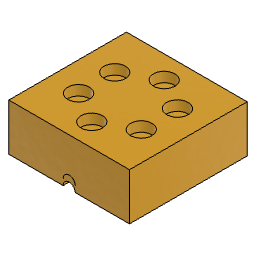
Tool change - six magnets (Autodesk Fusion 360 design; units mm, degrees)
Autodesk Fusion 360 part; units mm, degrees
note: some values were not read from the file. Set by a fixed rule: which sketch regions a step uses.
sketch "Sketch1" plane through (0, 0, 0) normal (0, 0, 1) x (1, 0, 0)
  line L0 (0, 1.3314) -> (42, 1.3314)
  line L1 (42, 1.3314) -> (42, 43.3314)
  line L2 (42, 43.3314) -> (0, 43.3314)
  line L3 (0, 43.3314) -> (0, 1.3314)
  dimension "d1" = 42
  dimension "d2" = 42
  constraint horizontal L0
  constraint vertical L1
  constraint horizontal L2
  constraint vertical L3
  measures "d1" distance of L0.start L2.end
  measures "d2" distance of L0.start L0.end
extrude "Extrude1" add sketch "Sketch1" along normal blind 7 makes body 1
sketch "Sketch2" plane through (0, 0, 7) normal (0, 0, 1) x (-1, 0, 0)
  line L0 (0, -43.3314) -> (0, -1.3314)
  line L1 (0, -1.3314) -> (-42, -1.3314)
  line L2 (-42, -1.3314) -> (-42, -43.3314)
  line L3 (-42, -43.3314) -> (0, -43.3314)
  circle A0 centre (-13, -22.3314) radius 3.55
  circle A1 centre (-29, -23.2838) radius 3.55
  dimension "d5" = 7.1
  dimension "d6" = 7.1
  dimension "d7" = 13
  dimension "d8" = 13
  dimension "d9" = 21
  measures "d5" diameter of A0
  measures "d6" diameter of A1
  measures "d7" distance of L0 A0.centre
  measures "d8" distance of L2 A1.centre
  measures "d9" distance of L1 A0.centre
sketch "Sketch4" plane through (0, 0, 7) normal (0, 0, 1) x (-1, 0, 0)
  line L0 (0, -43.3314) -> (0, -1.3314)
  line L1 (0, -1.3314) -> (-42, -1.3314)
  line L2 (-42, -1.3314) -> (-42, -43.3314)
  line L3 (-42, -43.3314) -> (0, -43.3314)
  circle A0 centre (-21, -22.3314) radius 3.55
  dimension "d12" = 7.1
  dimension "d13" = 21
  dimension "d14" = 21
  measures "d12" diameter of A0
  measures "d13" distance of L3 A0.centre
  measures "d14" distance of L0 A0.centre
extrude "Extrude3" cut sketch "Sketch4" against normal blind 3.3 contours A0 bodies 1
sketch "Sketch5" plane through (0, 0, 0) normal (0, 0, -1) x (1, 0, 0)
  line L0 (0, -1.3314) -> (0, -43.3314)
  line L1 (0, -43.3314) -> (42, -43.3314)
  line L2 (42, -43.3314) -> (42, -1.3314)
  line L3 (42, -1.3314) -> (0, -1.3314)
sketch "Sketch6" plane through (0, 0, 0) normal (0, 0, -1) x (1, 0, 0)
sketch "Sketch7" plane through (0, 0, 0) normal (0, 0, -1) x (1, 0, 0)
  line L0 (5.5, -6.1414) -> (36.5, -6.1414)
  line L1 (36.5, -6.1414) -> (36.5, -38.5214)
  line L2 (36.5, -38.5214) -> (5.5, -38.5214)
  line L3 (5.5, -38.5214) -> (5.5, -6.1414)
  line L4 (0, -1.3314) -> (0, -43.3314)
  line L5 (0, -43.3314) -> (42, -43.3314)
  line L6 (19, -6.1414) -> (23, -6.1414)
  line L7 (23, -6.1414) -> (23, -1)
  line L8 (23, -1) -> (19, -1)
  line L9 (19, -1) -> (19, -6.1414)
  line L10 (15.15, -38.5214) -> (26.85, -38.5214)
  line L11 (26.85, -38.5214) -> (26.85, -44)
  line L12 (26.85, -44) -> (15.15, -44)
  line L13 (15.15, -44) -> (15.15, -38.5214)
  line L14 (0, -1.3314) -> (42, -1.3314)
  line L15 (42, -1.3314) -> (42, -43.3314)
  line L16 (42, -43.3314) -> (0, -43.3314)
  line L17 (0, -43.3314) -> (0, -1.3314)
  dimension "d17" = 31
  dimension "d18" = 32.38
  dimension "d19" = 5.5
  dimension "d20" = 4.81
  dimension "d21" = 4
  dimension "d22" = 13.5
  dimension "d23" = 11.7
  dimension "d24" = 9.65
  constraint horizontal L0
  constraint vertical L1
  constraint horizontal L2
  constraint vertical L3
  constraint horizontal L6
  constraint vertical L7
  constraint horizontal L8
  constraint vertical L9
  constraint coincident L0 L6.start
  constraint horizontal L10
  constraint vertical L11
  constraint horizontal L12
  constraint vertical L13
  constraint coincident L2 L10.start
  constraint horizontal L14
  constraint vertical L15
  constraint horizontal L16
  constraint vertical L17
  constraint coincident L5.end L15.end
  constraint coincident L4.start L14.start
  measures "d17" distance of L0.start L0.end
  measures "d18" distance of L0.end L1.end
  measures "d19" distance of L3 L4
  measures "d20" distance of L2 L5
  measures "d21" distance of L7.end L8.end
  measures "d22" distance of L3 L9
  measures "d23" distance of L11.end L12.end
  measures "d24" distance of L3 L13
extrude "Extrude4" add sketch "Sketch7" along normal blind 6.55 contours L0 L2 L3 L4 L5 L9 L13 L14 L16 L17 | L0 L1 L2 L5 L7 L11 L14 L15 L16 bodies 1
sketch "Sketch8" plane through (0, 0, -6.55) normal (0, 0, -1) x (1, 0, 0)
  line L0 (15.15, -43.3314) -> (15.15, -38.5214)
  line L1 (15.15, -38.5214) -> (5.5, -38.5214)
  line L2 (5.5, -38.5214) -> (5.5, -6.1414)
  line L3 (5.5, -6.1414) -> (19, -6.1414)
  line L4 (19, -6.1414) -> (19, -1.3314)
  line L5 (19, -1.3314) -> (0, -1.3314)
  line L6 (0, -1.3314) -> (0, -43.3314)
  line L7 (0, -43.3314) -> (15.15, -43.3314)
sketch "Sketch9" plane through (0, 6.1414, 0) normal (0, 1, 0) x (-1, 0, 0)
  line L0 (-23, 0) -> (-36.5, 0)
  line L1 (-36.5, 0) -> (-36.5, -6.55)
  line L2 (-36.5, -6.55) -> (-23, -6.55)
  line L3 (-23, -6.55) -> (-23, 0)
sketch "Sketch10" plane through (0, 6.1414, 0) normal (0, 1, 0) x (-1, 0, 0)
  line L0 (-18.9881, 0) -> (-22.9881, 0)
  line L1 (-22.9881, 0) -> (-22.9881, -6.55)
  line L2 (-22.9881, -6.55) -> (-18.9881, -6.55)
  line L3 (-18.9881, -6.55) -> (-18.9881, 0)
  circle A0 centre (-20.9881, -6.55) radius 2
  dimension "d27" = 6.55
  dimension "d28" = 4
  dimension "d29" = 4
  constraint horizontal L0
  constraint vertical L1
  constraint horizontal L2
  constraint vertical L3
  constraint midpoint L2 A0.centre
  measures "d27" distance of L0.start L2.end
  measures "d28" distance of L1.end L2.end
  measures "d29" diameter of A0
sketch "Sketch11" plane through (0, 0, -6.55) normal (0, 0, -1) x (1, 0, 0)
  line L0 (23, -6.1414) -> (36.5, -6.1414)
  line L1 (36.5, -6.1414) -> (36.5, -38.5214)
  line L2 (36.5, -38.5214) -> (26.85, -38.5214)
  line L3 (26.85, -38.5214) -> (26.85, -43.3314)
  line L4 (26.85, -43.3314) -> (42, -43.3314)
  line L5 (42, -43.3314) -> (42, -1.3314)
  line L6 (42, -1.3314) -> (23, -1.3314)
  line L7 (23, -1.3314) -> (23, -6.1414)
extrude "Extrude11" add sketch "Sketch11" sketch "Sketch8" along normal blind 2 of sketch 2 bodies 1
sketch "Sketch20" plane through (0, 0, 0) normal (0, 0, -1) x (1, 0, 0)
sketch "Sketch21" plane through (0, 43.3314, 0) normal (0, 1, 0) x (-1, 0, 0)
  line L0 (-26.85, 0) -> (-15.15, 0)
  line L1 (-15.15, 0) -> (-15.15, -8.55)
  line L2 (-15.15, -8.55) -> (0, -8.55)
  line L3 (0, -8.55) -> (0, 7)
  line L4 (0, 7) -> (-42, 7)
  line L5 (-42, 7) -> (-42, -8.55)
  line L6 (-42, -8.55) -> (-26.85, -8.55)
  line L7 (-26.85, -8.55) -> (-26.85, 0)
  circle A0 centre (-21, -8) radius 5.85
  dimension "d62" = 11.7
  measures "d62" diameter of A0
extrude "Extrude12" add sketch "Sketch21" against normal blind 4.81 contours L0 L1 L7 A0 bodies 1
sketch "Sketch22" plane through (0, 1.3314, 0) normal (0, -1, 0) x (1, 0, 0)
  line L0 (19, 0) -> (23, 0)
  line L1 (23, 0) -> (23, -8.55)
  line L2 (23, -8.55) -> (42, -8.55)
  line L3 (42, -8.55) -> (42, 7)
  line L4 (42, 7) -> (0, 7)
  line L5 (0, 7) -> (0, -8.55)
  line L6 (0, -8.55) -> (19, -8.55)
  line L7 (19, -8.55) -> (19, 0)
  line L8 (23, -8.55) -> (19, -8.55)
  circle A0 centre (21, -8.55) radius 2
  dimension "d65" = 4
  constraint coincident L1.end L2.start
  constraint coincident L6.end L7.start
  constraint midpoint L8 A0.centre
  measures "d65" diameter of A0
extrude "Extrude13" add sketch "Sketch22" against normal blind 4.81 contours L0 L1 L7 A0 bodies 1
sketch "Sketch23" plane through (0, 6.1414, 0) normal (0, 1, 0) x (-1, 0, 0)
  line L0 (-5.5, 0) -> (-36.5, 0)
  line L1 (-36.5, 0) -> (-36.5, -8.55)
  line L2 (-36.5, -8.55) -> (-23, -8.55)
  arc A0 (-19, -8.55) -> (-23, -8.55) centre (-21, -8.55) ccw
  line L3 (-19, -8.55) -> (-5.5, -8.55)
  line L4 (-5.5, -8.55) -> (-5.5, 0)
sketch "Sketch12" plane through (0, 0, -6.55) normal (0, 0, -1) x (1, 0, 0)
extrude "Extrude5" add sketch "Sketch10" against normal blind 4.81 separate body contours L0 L1 L3 A0 makes body 2
sketch "Sketch14" plane through (0, 0, -6.55) normal (0, 0, -1) x (1, 0, 0)
sketch "Sketch15" plane through (0, 43.3314, 0) normal (0, 1, 0) x (-1, 0, 0)
  line L0 (-26.85, 0) -> (-15.15, 0)
  line L1 (-15.15, 0) -> (-15.15, -6.55)
  line L2 (-15.15, -6.55) -> (0, -6.55)
  line L3 (0, -6.55) -> (0, 7)
  line L4 (0, 7) -> (-42, 7)
  line L5 (-42, 7) -> (-42, -6.55)
  line L6 (-42, -6.55) -> (-26.85, -6.55)
  line L7 (-26.85, -6.55) -> (-26.85, 0)
  line L8 (-15.15, -6.55) -> (-26.85, -6.55)
  line L9 (-26.85, -6.55) -> (-26.85, 0)
  line L10 (-26.85, 0) -> (-15.15, 0)
  line L11 (-15.15, 0) -> (-15.15, -6.55)
  circle A0 centre (-21, -6.55) radius 5.85
  dimension "d32" = 11.7
  constraint horizontal L8
  constraint vertical L9
  constraint horizontal L10
  constraint vertical L11
  constraint coincident L0.start L7.end
  constraint coincident L1.end L2.start
  constraint midpoint L8 A0.centre
  measures "d32" diameter of A0
extrude "Extrude6" add sketch "Sketch15" against normal blind 4.81 contours L0 L1 L7 L9 L10 L11 A0 bodies 1
extrude "Extrude7" cut 1 faces at (20.9383, 1.3314, -1.5185) along direction (0, 1, 0) blind 6 on bodies 2 bodies 1 2
sketch "Sketch16" plane through (0, 1.3314, 0) normal (0, -1, 0) x (1, 0, 0)
  line L0 (18.9881, -6.55) -> (18.9881, 0)
  line L1 (18.9881, 0) -> (22.9881, 0)
  line L2 (42, -8.55) -> (42, 7)
  line L3 (42, 7) -> (0, 7)
  line L4 (0, 7) -> (0, -8.55)
  line L5 (23, -6.55) -> (18.9881, -6.55)
  line L6 (18.9881, -6.55) -> (18.9881, 0)
  line L7 (18.9881, 0) -> (23, 0)
  line L8 (23, 0) -> (23, -6.55)
  circle A0 centre (20.9941, -6.55) radius 2.006
  line L9 (22.9881, 0) -> (22.9881, -6.55)
  arc A1 (22.9881, -6.55) -> (18.9881, -6.55) centre (20.9881, -6.55) ccw
  arc A2 (23, -8.55) -> (19, -8.55) centre (21, -8.55) ccw
  line L10 (23, -8.55) -> (42, -8.55)
  line L11 (0, -8.55) -> (19, -8.55)
  dimension "d37" = 4.012
  constraint horizontal L5
  constraint vertical L6
  constraint horizontal L7
  constraint vertical L8
  constraint coincident L0.end L1.start
  constraint midpoint L5 A0.centre
  measures "d37" diameter of A0
extrude "Extrude8" add sketch "Sketch16" against normal blind 4.81 contours L0 L1 L6 L7 A0 L9 bodies 2 1
extrude "Extrude9" add 1 faces at (20.7445, 21.2299, 3.7) along direction (0, 0, 1) blind 3.3 on bodies 2 bodies 2
sketch "Sketch17" plane through (0, 0, 7) normal (0, 0, 1) x (-1, 0, 0)
  line L0 (0, -43.3314) -> (0, -1.3314)
  line L1 (0, -1.3314) -> (-42, -1.3314)
  line L2 (-42, -1.3314) -> (-42, -43.3314)
  line L3 (-42, -43.3314) -> (0, -43.3314)
sketch "Sketch18" plane through (0, 0, 7) normal (0, 0, 1) x (-1, 0, 0)
  circle A0 centre (-21, -10.3314) radius 3.55
  circle A1 centre (-31.3924, -16.3314) radius 3.55
  circle A2 centre (-31.3933, -28.3314) radius 3.55
  circle A3 centre (-21, -34.3314) radius 3.55
  circle A4 centre (-10.6087, -16.3314) radius 3.55
  circle A5 centre (-10.6078, -28.3314) radius 3.55
  line L0 (0, -1.3314) -> (-42, -1.3314)
  line L1 (-42, -1.3314) -> (-42, -43.3314)
  line L2 (-21, -1.3314) -> (-21, -43.3314) construction
  line L3 (-42, -43.3314) -> (0, -43.3314) construction
  line L4 (-42, -22.3314) -> (0, -22.3314) construction
  line L5 (-42, -34.4552) -> (-0.5498, -10.5239) construction
  line L6 (-42, -10.2071) -> (2.5417, -35.9233) construction
  dimension "d42" = 7.1
  dimension "d43" = 7.1
  dimension "d44" = 7.1
  dimension "d45" = 7.1
  dimension "d46" = 7.1
  dimension "d47" = 7.1
  dimension "d48" = 24
  dimension "d49" = 24
  dimension "d50" = 24
  dimension "d51" = 9
  dimension "d54" = 60
  dimension "d55" = 60
  dimension "d56" = 6
  dimension "d57" = 6
  constraint midpoint L0 L2.start
  constraint perpendicular L0 L2
  constraint coincident L2.end L3
  constraint coincident A0.centre L2
  constraint coincident A3.centre L2
  constraint midpoint L1 L4.start
  constraint perpendicular L1 L4
  constraint coincident L1 L5.start
  constraint coincident L1 L6.start
  constraint coincident A4.centre L5
  constraint coincident A2.centre L5
  constraint coincident A5.centre L6
  constraint coincident A1.centre L6
  measures "d42" diameter of A0
  measures "d43" diameter of A1
  measures "d44" diameter of A2
  measures "d45" diameter of A3
  measures "d46" diameter of A4
  measures "d47" diameter of A5
  measures "d48" vertical distance of A0.centre A3.centre
  measures "d49" distance of A2.centre A4.centre
  measures "d50" distance of A1.centre A5.centre
  measures "d51" distance of A0.centre L0
  measures "d54" angle of L2 L5
  measures "d55" angle of L2 L6
  measures "d56" distance of A4.centre L4
  measures "d57" distance of A1.centre L4
extrude "Extrude10" cut sketch "Sketch18" against normal blind 3.3 bodies 2
sketch "Sketch19" plane through (0, 0, 7) normal (0, 0, 1) x (-1, 0, 0)
  line L0 (-31.3619, -16.3554) -> (-20.9754, -10.3528)
  line L1 (-20.9754, -10.3528) -> (-10.5888, -16.3554)
  line L2 (-10.5888, -16.3554) -> (-10.5888, -28.428)
  line L3 (-10.5888, -28.428) -> (-20.9248, -34.4014)
  line L4 (-20.9248, -34.4014) -> (-31.2607, -28.428)
  line L5 (-31.2607, -28.428) -> (-20.9248, -28.8672)
  constraint vertical L2
  constraint parallel L0 L3
  constraint parallel L1 L4
sketch "Sketch13" plane through (0, 0, -6.55) normal (0, 0, -1) x (1, 0, 0)
sketch "Sketch24" plane through (21, 6.1414, -4.275) normal (0, 1, 0) x (-1, 0, 0)
sketch "Sketch25" plane through (0, 0, 0) normal (0, 0, -1) x (1, 0, 0)
extrude "Extrude14" cut 1 faces at (0, 29.3314, -3.3667) along direction (1, 0, 0) blind 2 on bodies 2 bodies 2
extrude "Extrude15" cut 1 faces at (42, 29.3314, 1.8167) along direction (-1, 0, 0) blind 2 on bodies 2 bodies 2
extrude "Extrude16" cut 1 faces at (6.5764, 43.3314, -2.3373) along direction (0, -1, 0) blind 1 on bodies 2 bodies 2
extrude "Extrude17" cut 1 faces at (21.0098, 1.3314, 3.1519) along direction (0, 1, 0) blind 1 on bodies 2 bodies 2
sketch "Sketch26" plane through (0, 0, -8.55) normal (0, 0, -1) x (1, 0, 0)
  line L0 (19, -2.3314) -> (2, -2.3314)
  line L1 (2, -2.3314) -> (2, -42.3314)
  line L2 (2, -42.3314) -> (15.15, -42.3314)
  line L3 (15.15, -42.3314) -> (15.15, -38.5214)
  line L4 (15.15, -38.5214) -> (5.5, -38.5214)
  line L5 (5.5, -38.5214) -> (5.5, -6.1414)
  line L6 (5.5, -6.1414) -> (19, -6.1414)
  line L7 (19, -6.1414) -> (19, -2.3314)
extrude "Extrude18" cut 1 faces at (21.0098, 2.3314, 3.1519) along direction (0, 1, 0) blind 0.5 on bodies 2 bodies 2
extrude "Extrude19" cut 1 faces at (6.5764, 42.3314, -2.3373) along direction (0, -1, 0) blind 0.5 on bodies 2 bodies 2
extrude "Extrude20" cut 1 faces at (21.0098, 2.8314, 3.1519) along direction (0, 1, 0) blind 1 on bodies 2 bodies 2
extrude "Extrude21" cut 1 faces at (40, 16.4981, -3.3667) along direction (-1, 0, 0) blind 1 on bodies 2 bodies 2
extrude "Extrude22" cut 1 faces at (6.5764, 41.8314, -2.3373) along direction (0, -1, 0) blind 1 on bodies 2 bodies 2
extrude "Extrude23" cut 1 faces at (2, 28.4981, 1.8167) along direction (1, 0, 0) blind 1 on bodies 2 bodies 2
sketch "Sketch27" plane through (0, 0, -8.55) normal (0, 0, -1) x (1, 0, 0)
  line L0 (3, -3.8314) -> (3, -40.8314)
  line L1 (3, -40.8314) -> (15.15, -40.8314)
  line L2 (15.15, -40.8314) -> (15.15, -38.5214)
  line L3 (15.15, -38.5214) -> (5.5, -38.5214)
  line L4 (5.5, -38.5214) -> (5.5, -6.1414)
  line L5 (5.5, -6.1414) -> (19, -6.1414)
  line L6 (19, -6.1414) -> (19, -3.8314)
  line L7 (19, -3.8314) -> (3, -3.8314)
sketch "Sketch28" plane through (0, 0, -8.55) normal (0, 0, -1) x (1, 0, 0)
  line L0 (3, -3.8314) -> (3, -40.8314)
  line L1 (3, -40.8314) -> (15.15, -40.8314)
  line L2 (15.15, -40.8314) -> (15.15, -38.5214)
  line L3 (15.15, -38.5214) -> (5.5, -38.5214)
  line L4 (5.5, -38.5214) -> (5.5, -6.1414)
  line L5 (5.5, -6.1414) -> (19, -6.1414)
  line L6 (19, -6.1414) -> (19, -3.8314)
  line L7 (19, -3.8314) -> (3, -3.8314)
extrude "Extrude24" add 1 faces at (21.0098, 3.8314, 3.1519) along direction (0, -1, 0) blind 1 on bodies 2 bodies 2
extrude "Extrude25" add 1 faces at (20.8543, 40.8314, 3.9445) along direction (0, 1, 0) blind 1 on bodies 2 bodies 2
extrude "Extrude26" add 1 faces at (39, 15.8314, 1.8167) along direction (1, 0, 0) blind 2 on bodies 2 bodies 2
extrude "Extrude27" add 1 faces at (3, 15.8314, 1.8167) along direction (-1, 0, 0) blind 2 on bodies 2 bodies 2
sketch "Sketch29" plane through (0, 0, -8.55) normal (0, 0, -1) x (1, 0, 0)
  line L0 (1, -41.8314) -> (15.15, -41.8314)
  line L1 (15.15, -41.8314) -> (15.15, -38.5214)
  line L2 (15.15, -38.5214) -> (5.5, -38.5214)
  line L3 (5.5, -38.5214) -> (5.5, -6.1414)
  line L4 (5.5, -6.1414) -> (19, -6.1414)
  line L5 (19, -6.1414) -> (19, -2.8314)
  line L6 (19, -2.8314) -> (1, -2.8314)
  line L7 (1, -2.8314) -> (1, -41.8314)
extrude "Extrude2" [suppressed]
sketch "Sketch3" plane through (0, 0, 7) normal (0, 0, 1) x (-1, 0, 0)
  circle A0 centre (-13, -22.3314) radius 3.55
  circle A1 centre (-29, -23.2838) radius 3.55
  line L0 (0, -43.3314) -> (0, -1.3314)
  line L1 (0, -1.3314) -> (-42, -1.3314)
  line L2 (-42, -1.3314) -> (-42, -43.3314)
  line L3 (-42, -43.3314) -> (0, -43.3314)
